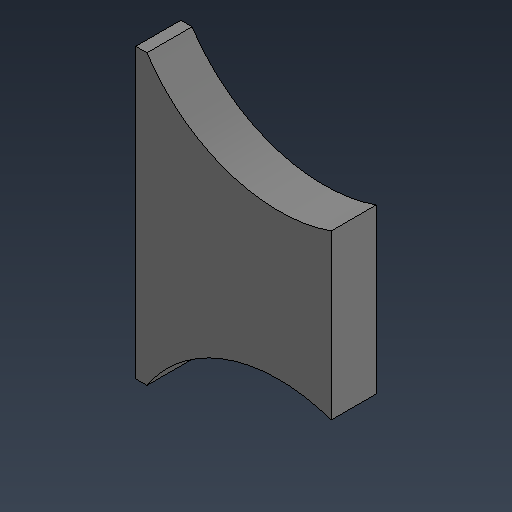
# Autodesk Inventor part: GearboxBearingHolderCover
Saved by Autodesk Inventor 2026.2 (Build 302298010, 298A)
## iProperties
Created: 2026-04-14
Part Number: GearboxBearingHolderCover
Material: Generic
Document SubType Name: Modeling
Designer: szymo
Density: 1 g/cm^3
Appearance: Default(1)
Author: szymo
Autodesk Inventor part; units mm, degrees
ref_plane "YZ Plane" through (0, 0, 0) normal (1, 0, 0) x (0, 1, 0)
ref_plane "XZ Plane" through (0, 0, 0) normal (0, 1, 0) x (-1, 0, 0)
ref_plane "XY Plane" through (0, 0, 0) normal (0, 0, 1) x (1, 0, 0)
sketch "Sketch1" plane through (0, 0, 0) normal (0, 0, 1) x (1, 0, 0)
  line L0 (3, -22.3883) -> (2, -22.3883)
  line L1 (2, -22.3883) -> (2, -47.9488)
  line L2 (2, -47.9488) -> (3, -47.9488)
  circle A0 centre (14.7, -14.7) radius 14
  circle A1 centre (14.7, -55.6371) radius 14
  circle A2 centre (14.7, -14.7) radius 14.7 construction
  line L3 (0, -14.7) -> (0, -55.6371) construction
  circle A3 centre (14.7, -55.6371) radius 14.7 construction
  circle A4 centre (12.35, -35.2722) radius 5
  line L4 (19.35, -27.9052) -> (19.35, -42.4319)
  circle A5 centre (14.7, -14.7) radius 14.7 projected
  circle A6 centre (14.7, -14.7) radius 14 projected
  circle A7 centre (14.7, -55.6371) radius 14.7 projected
  circle A8 centre (14.7, -55.6371) radius 14 projected
  circle A9 centre (12.35, -35.2722) radius 3.2 construction
  circle A10 centre (12.35, -35.2722) radius 4.8 construction
  point P0 (0, 0)
  dimension "d0" = 2
  dimension "d2" = 2
  dimension "d5" = 10
  dimension "d6" = 1
  dimension "d7" = 1
  constraints: 10 end point, 5 coincident, 4 point on circle, 3 centre point, 3 vertical, 2 concentric, 2 horizontal alignment, 2 perpendicular, 1 horizontal, 6 other
  measures "d0" distance between parallel lines of L3 L1
  measures "d2" distance edge to line of A4 L4
  measures "d5" diameter of A4
  measures "d6" distance of L0.start L0.end
  measures "d7" distance of L1.end L2.end
ref_plane "Work Plane1" through (5.5618, -42.0604, 3.6) normal (0, 0, 1) x (0.7075365, 0.7066768, 0)
extrude "Extrusion1" add sketch "Sketch1" along normal up to surface (3.6 mm away) contours A0 L4 A5 L0 | A5 L4 A7 L2 L1 L0 | L4 A1 L2 A7 picked at (4.054, -24.0446) picked at (4.054, -46.2925)
sketch "Sketch2" plane through (2, -47.9488, 3.6) normal (0, 0, 1) x (1, 0, 0)
  circle A0 centre (10.35, 12.6766) radius 5 projected
  line L0 (0, 0) -> (0, 25.5605) projected
  line L1 (1, 0) -> (0, 0) projected
  arc A1 (17.35, 5.5169) -> (1, 0) centre (12.7, -7.6883) ccw projected
  line L2 (17.35, 20.0436) -> (17.35, 5.5169) projected
  arc A2 (1, 25.5605) -> (17.35, 20.0436) centre (12.7, 33.2488) ccw projected
  line L3 (0, 25.5605) -> (1, 25.5605) projected
  point P0 (-2, 47.9488)
extrude "Extrusion2" add sketch "Sketch2" along normal blind 0.4 contours A0 | L0 L3 A2 L2 A1 L1
sketch "Sketch3" plane through (2, -47.9488, 0) normal (-1, 0, 0) x (0, 0, 1)
  line L0 (0, 25.5605) -> (4, 25.5605) projected
  line L1 (0, 25.5605) -> (0, 0) projected
  line L2 (0, 0) -> (4, 0) projected
  line L3 (4, 25.5605) -> (4, 0) projected
  line L4 (4, 12.7802) -> (0, 12.7802) construction
  circle A0 centre (2, 17.7802) radius 2
  circle A1 centre (2, 7.7802) radius 2
  line L5 (0, 17.6766) -> (0, 7.6766) projected
  line L6 (0, 15.7802) -> (4, 15.7802) construction
  line L7 (0, 9.7802) -> (4, 9.7802) construction
  point P0 (0, 47.9488)
  dimension "d10" = 3
  dimension "d11" = 3
  constraints: 6 end point, 6 tangent, 4 point on line, 2 centre point, 2 midpoint, 2 perpendicular
  measures "d10" distance between parallel lines of L4 L7
  measures "d11" distance between parallel lines of L6 L4
hole "Hole1" at (2, -30.1685, 2) at (2, -40.1685, 2) direction (1, 0, 0) diameter 3 depth 5.5 counterbore diameter 3.5 counterbore depth 0.5
equation "\"d10\" = d11"
body "Solid1"
